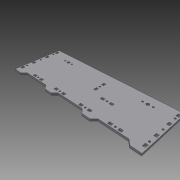
# Autodesk Inventor part: front
Saved by Autodesk Inventor 2014 (Build 180170000, 170)
## iProperties
Created: 2013-12-05
Part Number: front
Material: Generic
Document SubType Name: Modeling
Designer: buben
Density: 1 g/cm^3
Appearance: Anodized - Dark Gray
Author: buben
Subject: Laser Cutted
Autodesk Inventor part; units mm, degrees
ref_plane "YZ Plane" through (0, 0, 0) normal (1, 0, 0) x (0, 1, 0)
ref_plane "XZ Plane" through (0, 0, 0) normal (0, 1, 0) x (-1, 0, 0)
ref_plane "XY Plane" through (0, 0, 0) normal (0, 0, 1) x (1, 0, 0)
sketch "Sketch1" plane through (0, 0, 0) normal (0, 0, 1) x (1, 0, 0)
  line L0 (0, 0) -> (353, 0)
  line L1 (353, 0) -> (353, 120)
  line L2 (353, 120) -> (0, 120)
  line L3 (0, 120) -> (0, 0)
  dimension "d0" = 120
  dimension "d1" = 353
  constraints: 8 end point, 2 parallel, 1 horizontal, 1 perpendicular
  measures "d0" distance of L2.end L0.start
  measures "d1" distance of L0.start L0.end
extrude "Extrusion1" add sketch "Sketch1" along normal blind 6
sketch "Sketch3" plane through (0, 0, 6) normal (0, 0, 1) x (1, 0, 0)
  line L0 (0, 0) -> (353, 0) projected
  line L1 (353, 120) -> (0, 120) projected
  line L2 (0, 120) -> (0, 0) projected
  circle A0 centre (63.5, 96) radius 4
  circle A1 centre (289.5, 96) radius 4
  line L3 (63.5, 96) -> (289.5, 96) construction
  point P0 (176.5, 96)
  point P1 (176.5, 120)
  dimension "d9" = 8
  dimension "d10" = 96
  dimension "d11" = 226
  constraints: 2 centre point, 2 end point, 2 midpoint, 1 equal radius, 1 horizontal alignment, 1 perpendicular, 1 vertical alignment
  measures "d9" diameter of A0
  measures "d10" distance from line of L0 L3.start
  measures "d11" distance of L3.start L3.end
extrude "Extrusion3" cut sketch "Sketch3" against normal through all
sketch "Sketch4" plane through (0, 0, 6) normal (0, 0, 1) x (1, 0, 0)
  line L0 (0, 0) -> (353, 0) projected
  line L1 (353, 120) -> (0, 120) projected
  line L2 (0, 120) -> (0, 0) projected
  circle A0 centre (6, 18.5) radius 2.25
  circle A1 centre (6, 57.5) radius 2.25
  circle A2 centre (6, 96.5) radius 2.25
  line L3 (176.5, 120) -> (176.5, 0) construction
  line L4 (3, 112) -> (9, 112)
  line L5 (9, 112) -> (9, 104)
  line L6 (9, 104) -> (3, 104)
  line L7 (3, 104) -> (3, 112)
  line L8 (3, 81) -> (9, 81)
  line L9 (9, 81) -> (9, 73)
  line L10 (9, 73) -> (3, 73)
  line L11 (3, 73) -> (3, 81)
  line L12 (3, 42) -> (9, 42)
  line L13 (9, 42) -> (9, 34)
  line L14 (9, 34) -> (3, 34)
  line L15 (3, 34) -> (3, 42)
  line L16 (3, 11) -> (9, 11)
  line L17 (9, 11) -> (9, 3)
  line L18 (9, 3) -> (3, 3)
  line L19 (3, 3) -> (3, 11)
  line L20 (6, 18.5) -> (6, 57.5) construction
  line L21 (6, 57.5) -> (6, 96.5) construction
  circle A3 centre (347, 18.5) radius 2.25
  circle A4 centre (347, 57.5) radius 2.25
  circle A5 centre (347, 96.5) radius 2.25
  line L22 (350, 112) -> (344, 112)
  line L23 (344, 112) -> (344, 104)
  line L24 (344, 104) -> (350, 104)
  line L25 (350, 104) -> (350, 112)
  line L26 (350, 81) -> (344, 81)
  line L27 (344, 81) -> (344, 73)
  line L28 (344, 73) -> (350, 73)
  line L29 (350, 73) -> (350, 81)
  line L30 (350, 42) -> (344, 42)
  line L31 (344, 42) -> (344, 34)
  line L32 (344, 34) -> (350, 34)
  line L33 (350, 34) -> (350, 42)
  line L34 (350, 11) -> (344, 11)
  line L35 (344, 11) -> (344, 3)
  line L36 (344, 3) -> (350, 3)
  line L37 (350, 3) -> (350, 11)
  line L38 (347, 18.5) -> (347, 57.5) construction
  line L39 (347, 57.5) -> (347, 96.5) construction
  point P0 (6, 104)
  point P1 (3, 38)
  point P2 (6, 38)
  point P3 (3, 77)
  point P4 (6, 77)
  point P5 (347, 104)
  point P6 (350, 38)
  point P7 (347, 38)
  point P8 (350, 77)
  point P9 (347, 77)
  dimension "d14" = 18.5
  dimension "d15" = 39
  dimension "d16" = 39
  dimension "d17" = 4.5
  dimension "d18" = 6
  dimension "d19" = 8
  dimension "d20" = 8
  dimension "d21" = 8
  dimension "d22" = 8
  dimension "d23" = 3
  dimension "d27" = 23
  dimension "d28" = 3
  constraints: 74 end point, 24 symmetric about line, 9 parallel, 7 collinear, 7 midpoint, 6 centre point, 4 horizontal, 4 perpendicular, 3 vertical alignment, 2 equal radius, 2 horizontal alignment, 3 other
  measures "d14" distance from line of L0 L20.start
  measures "d15" distance of L20.start L20.end
  measures "d16" distance of L20.end L21.end
  measures "d17" diameter of A0
  measures "d18" distance of L4.start L4.end
  measures "d19" distance of L6.end L4.start
  measures "d20" distance of L10.end L8.start
  measures "d21" distance of L14.end L12.start
  measures "d22" distance of L18.end L16.start
  measures "d23" distance between parallel lines of L0 L18
  measures "d27" distance between parallel lines of L8 L6
  measures "d28" distance between parallel lines of L2 L7
extrude "Extrusion4" cut sketch "Sketch4" against normal through all
sketch "Sketch5" plane through (0, 0, 6) normal (0, 0, 1) x (1, 0, 0)
  line L0 (0, 0) -> (353, 0) projected
  line L1 (51.2, 9) -> (59.2, 9)
  line L2 (59.2, 9) -> (59.2, 3)
  line L3 (59.2, 3) -> (51.2, 3)
  line L4 (51.2, 3) -> (51.2, 9)
  line L5 (74.2, 9) -> (82.2, 9)
  line L6 (82.2, 9) -> (82.2, 3)
  line L7 (82.2, 3) -> (74.2, 3)
  line L8 (74.2, 3) -> (74.2, 9)
  line L9 (59.2, 9) -> (74.2, 3) construction
  line L10 (74.2, 9) -> (59.2, 3) construction
  circle A0 centre (66.7, 6) radius 2.25
  line L11 (124.4, 9) -> (132.4, 9)
  line L12 (132.4, 9) -> (132.4, 3)
  line L13 (132.4, 3) -> (124.4, 3)
  line L14 (124.4, 3) -> (124.4, 9)
  line L15 (147.4, 9) -> (155.4, 9)
  line L16 (155.4, 9) -> (155.4, 3)
  line L17 (155.4, 3) -> (147.4, 3)
  line L18 (147.4, 3) -> (147.4, 9)
  line L19 (132.4, 9) -> (147.4, 3) construction
  line L20 (147.4, 9) -> (132.4, 3) construction
  circle A1 centre (139.9, 6) radius 2.25
  line L21 (197.6, 9) -> (205.6, 9)
  line L22 (205.6, 9) -> (205.6, 3)
  line L23 (205.6, 3) -> (197.6, 3)
  line L24 (197.6, 3) -> (197.6, 9)
  line L25 (220.6, 9) -> (228.6, 9)
  line L26 (228.6, 9) -> (228.6, 3)
  line L27 (228.6, 3) -> (220.6, 3)
  line L28 (220.6, 3) -> (220.6, 9)
  line L29 (205.6, 9) -> (220.6, 3) construction
  line L30 (220.6, 9) -> (205.6, 3) construction
  circle A2 centre (213.1, 6) radius 2.25
  line L31 (270.8, 9) -> (278.8, 9)
  line L32 (278.8, 9) -> (278.8, 3)
  line L33 (278.8, 3) -> (270.8, 3)
  line L34 (270.8, 3) -> (270.8, 9)
  line L35 (293.8, 9) -> (301.8, 9)
  line L36 (301.8, 9) -> (301.8, 3)
  line L37 (301.8, 3) -> (293.8, 3)
  line L38 (293.8, 3) -> (293.8, 9)
  line L39 (278.8, 9) -> (293.8, 3) construction
  line L40 (293.8, 9) -> (278.8, 3) construction
  circle A3 centre (286.3, 6) radius 2.25
  line L41 (51.2, 6) -> (9, 6) construction
  line L42 (82.2, 6) -> (124.4, 6) construction
  line L43 (155.4, 6) -> (197.6, 6) construction
  line L44 (228.6, 6) -> (270.8, 6) construction
  line L45 (301.8, 6) -> (344, 6) construction
  point P0 (9, 3)
  point P1 (344, 3)
  point P2 (286.3, 6)
  dimension "d31" = 8
  dimension "d32" = 6
  dimension "d33" = 8
  dimension "d34" = 15
  dimension "d35" = 4.5
  dimension "d36" = 8
  dimension "d37" = 6
  dimension "d38" = 8
  dimension "d39" = 15
  dimension "d40" = 4.5
  dimension "d41" = 8
  dimension "d42" = 6
  dimension "d43" = 8
  dimension "d44" = 15
  dimension "d45" = 4.5
  dimension "d46" = 8
  dimension "d47" = 6
  dimension "d48" = 8
  dimension "d49" = 15
  dimension "d50" = 4.5
  dimension "d51" = 3
  constraints: 90 end point, 17 parallel, 13 collinear, 13 midpoint, 8 horizontal, 8 perpendicular, 4 centre point, 3 horizontal alignment, 2 vertical alignment
  measures "d31" distance of L1.start L1.end
  measures "d32" distance of L3.end L1.start
  measures "d33" distance of L5.start L5.end
  measures "d34" distance between parallel lines of L8 L2
  measures "d35" diameter of A0
  measures "d36" distance of L14.end L11.end
  measures "d37" distance of L14.start L14.end
  measures "d38" distance of L20.start L15.end
  measures "d39" distance between parallel lines of L18 L12
  measures "d40" diameter of A1
  measures "d41" distance of L24.end L21.end
  measures "d42" distance of L24.start L24.end
  measures "d43" distance of L30.start L25.end
  measures "d44" distance between parallel lines of L28 L22
  measures "d45" diameter of A2
  measures "d46" distance of L34.end L31.end
  measures "d47" distance of L34.start L34.end
  measures "d48" distance of L40.start L35.end
  measures "d49" distance between parallel lines of L38 L32
  measures "d50" diameter of A3
  measures "d51" distance between parallel lines of L0 L3
extrude "Extrusion5" cut sketch "Sketch5" against normal through all
sketch "Sketch6" plane through (0, 0, 6) normal (0, 0, 1) x (1, 0, 0)
  line L0 (0, 0) -> (353, 0) projected
  line L1 (0, 120) -> (0, 0) projected
  line L2 (0, 0) -> (0, -10)
  line L3 (0, -10) -> (23, -10)
  line L4 (23, -10) -> (33, 0)
  line L5 (102, 0) -> (112, -10)
  line L6 (112, -10) -> (132, -10)
  line L7 (132, -10) -> (142, 0)
  line L8 (211, 0) -> (221, -10)
  line L9 (221, -10) -> (241, -10)
  line L10 (241, -10) -> (251, 0)
  line L11 (353, 0) -> (353, -10)
  line L12 (353, -10) -> (330, -10)
  line L13 (330, -10) -> (320, 0)
  line L14 (23, -10) -> (112, -10) construction
  line L15 (132, -10) -> (221, -10) construction
  line L16 (241, -10) -> (330, -10) construction
  dimension "d54" = 20
  dimension "d55" = 23
  dimension "d56" = 45
  dimension "d57" = 10
  constraints: 30 end point, 13 collinear, 8 perpendicular, 6 point on line
  measures "d54" distance of L5.end L6.end
  measures "d55" distance of L2.end L3.end
  measures "d56" angle of L4 L3
  measures "d57" distance of L0.start L2.end
extrude "Extrusion6" add sketch "Sketch6" against normal blind 6
sketch "Sketch7" plane through (0, 0, 6) normal (0, 0, 1) x (1, 0, 0)
  line L0 (147.4, 9) -> (155.4, 9) projected
  line L1 (353, 120) -> (0, 120) projected
  line L2 (173.5, 81.1) -> (179.5, 81.1) construction
  line L3 (179.5, 81.1) -> (179.5, 68.88) construction
  line L4 (179.5, 68.88) -> (173.5, 68.88) construction
  line L5 (173.5, 68.88) -> (173.5, 81.1) construction
  line L6 (182.5, 90.49) -> (188.5, 90.49)
  line L7 (188.5, 90.49) -> (188.5, 82.49)
  line L8 (188.5, 82.49) -> (182.5, 82.49)
  line L9 (182.5, 82.49) -> (182.5, 90.49)
  line L10 (182.5, 67.49) -> (188.5, 67.49)
  line L11 (188.5, 67.49) -> (188.5, 59.49)
  line L12 (188.5, 59.49) -> (182.5, 59.49)
  line L13 (182.5, 59.49) -> (182.5, 67.49)
  line L14 (182.5, 82.49) -> (188.5, 67.49) construction
  line L15 (182.5, 67.49) -> (188.5, 82.49) construction
  circle A0 centre (185.5, 74.99) radius 2.25
  line L16 (213.5, 51.49) -> (221.5, 51.49)
  line L17 (221.5, 51.49) -> (221.5, 45.49)
  line L18 (221.5, 45.49) -> (213.5, 45.49)
  line L19 (213.5, 45.49) -> (213.5, 51.49)
  line L20 (236.5, 51.49) -> (244.5, 51.49)
  line L21 (244.5, 51.49) -> (244.5, 45.49)
  line L22 (244.5, 45.49) -> (236.5, 45.49)
  line L23 (236.5, 45.49) -> (236.5, 51.49)
  line L24 (221.5, 45.49) -> (236.5, 51.49) construction
  line L25 (221.5, 51.49) -> (236.5, 45.49) construction
  circle A1 centre (229, 48.49) radius 2.25
  point P0 (0, 0)
  point P1 (185.5, 74.99)
  point P2 (179.5, 74.99)
  point P3 (176.5, 81.1)
  point P4 (176.5, 120)
  dimension "d60" = 12.22
  dimension "d61" = 6
  dimension "d62" = 72.1
  dimension "d63" = 6
  dimension "d64" = 8
  dimension "d65" = 15
  dimension "d66" = 4.5
  dimension "d67" = 3
  dimension "d68" = 8
  dimension "d69" = 8
  dimension "d70" = 8
  dimension "d71" = 6
  dimension "d72" = 25
  dimension "d73" = 15
  dimension "d74" = 8
  constraints: 48 end point, 10 parallel, 6 midpoint, 5 horizontal, 5 perpendicular, 4 collinear, 2 centre point, 1 equal radius, 1 horizontal alignment, 1 vertical alignment
  measures "d60" distance of L4.end L2.start
  measures "d61" distance of L2.start L2.end
  measures "d62" distance between parallel lines of L0 L2
  measures "d63" distance of L6.start L6.end
  measures "d64" distance of L8.end L6.start
  measures "d65" distance between parallel lines of L10 L8
  measures "d66" diameter of A0
  measures "d67" distance between parallel lines of L3 L9
  measures "d68" distance of L10.end L11.end
  measures "d69" distance of L16.start L16.end
  measures "d70" distance of L20.start L20.end
  measures "d71" distance of L18.end L16.start
  measures "d72" distance from line of L16.start L11
  measures "d73" distance between parallel lines of L23 L17
  measures "d74" distance between parallel lines of L12 L16
extrude "Extrusion7" cut sketch "Sketch7" against normal through all
sketch "Sketch8" plane through (0, 0, 6) normal (0, 0, 1) x (1, 0, 0)
  line L0 (213.5, 51.49) -> (221.5, 51.49) projected
  circle A0 centre (63.5, 96) radius 4 projected
  circle A1 centre (289.5, 96) radius 4 projected
  line L1 (0, -10) -> (23, -10) projected
  circle A2 centre (51.5, 96) radius 2.25
  circle A3 centre (75.5, 96) radius 2.25
  circle A4 centre (277.5, 96) radius 2.25
  circle A5 centre (301.5, 96) radius 2.25
  line L2 (51.5, 96) -> (75.5, 96) construction
  line L3 (277.5, 96) -> (301.5, 96) construction
  point P0 (0, 0)
  dimension "d77" = 24
  dimension "d78" = 4.5
  constraints: 4 centre point, 4 end point, 3 equal radius, 2 coincident, 2 collinear, 2 midpoint, 2 parallel
  measures "d77" distance of L2.start L2.end
  measures "d78" diameter of A2
extrude "Extrusion8" cut sketch "Sketch8" against normal through all contours A2 | A3 | A4 | A5
body "Solid1"
